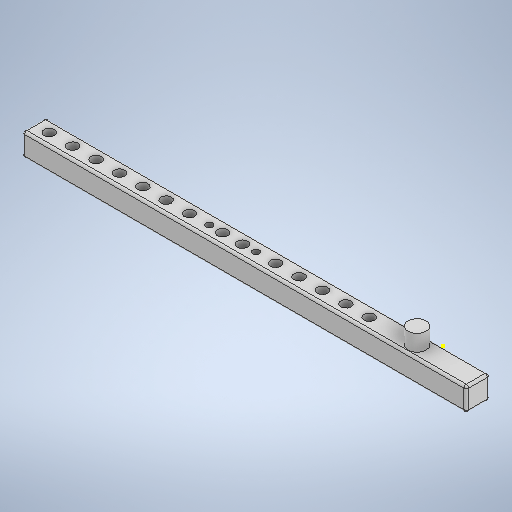
# Autodesk Inventor part: brazo apoyo
Saved by Autodesk Inventor 2025.2 (Build 292293000, 293)
## iProperties
Created: 2025-03-30
Part Number: brazo apoyo
Material: Generic
Document SubType Name: Modeling
Designer: maqmat
Density: 1 g/cm^3
Appearance: Default
Author: maqmat
Autodesk Inventor part; units mm, degrees
ref_plane "YZ Plane" through (0, 0, 0) normal (1, 0, 0) x (0, 1, 0)
ref_plane "XZ Plane" through (0, 0, 0) normal (0, 1, 0) x (-1, 0, 0)
ref_plane "XY Plane" through (0, 0, 0) normal (0, 0, 1) x (1, 0, 0)
sketch "Sketch1" plane through (0, 0, 0) normal (0, 1, 0) x (-1, 0, 0)
  line L0 (0, 0) -> (170, 0)
  line L1 (170, 0) -> (170, 10)
  line L2 (170, 10) -> (0, 10)
  line L3 (0, 10) -> (0, 0)
  dimension "d0" = 170
  dimension "d1" = 10
  constraints: 8 end point, 2 parallel, 1 horizontal, 1 perpendicular
  measures "d0" distance of L2.end L1.end
  measures "d1" distance of L1.end L0.end
extrude "Extrusion1" add sketch "Sketch1" along normal blind 10
sketch "Sketch2" plane through (0, 10, 0) normal (0, 1, 0) x (1, 0, 0)
  line L0 (0, -10) -> (0, 0) projected
  line L1 (0, -5) -> (-2.2, -5)
  circle A0 centre (-6.1, -5) radius 3.9
  line L2 (0, 0) -> (-170, 0) projected
  line L3 (-170, -10) -> (0, -10) projected
  circle A1 centre (-75, -5) radius 1.5
  circle A2 centre (-95, -5) radius 1.5
  dimension "d35" = 10
  dimension "d4" = 2.2
  dimension "d8" = 3
  dimension "d9" = 3
  constraints: 2 centre point, 2 end point, 1 horizontal, 1 horizontal alignment, 1 midpoint, 2 other
  measures "d4" distance of L1.start L1.end
  measures "d8" diameter of A1
  measures "d9" diameter of A2
extrude "Extrusion2" cut sketch "Sketch2" against normal blind 10 contours A1
extrude "Extrusion3" cut sketch "Sketch2" against normal blind 10 contours A2
extrude "Extrusion4" add sketch "Sketch2" along normal blind 7 contours A0
sketch "Sketch3" plane through (0, 10, 0) normal (0, 1, 0) x (1, 0, 0)
  line L0 (-170, 0) -> (-170, -10) projected
  line L1 (-170, -5) -> (-10, -5)
  circle A0 centre (-6.1, -5) radius 3.9 projected
  line L2 (-165.7, -5) -> (-163.45, -5)
  circle A1 centre (-163.45, -5) radius 2.25
  circle A2 centre (-153.45, -5) radius 2.25
  circle A3 centre (-143.45, -5) radius 2.25
  circle A4 centre (-133.45, -5) radius 2.25
  circle A5 centre (-123.45, -5) radius 2.25
  circle A6 centre (-113.45, -5) radius 2.25
  circle A7 centre (-103.45, -5) radius 2.25
  circle A8 centre (-95, -5) radius 1.5 projected
  line L3 (-93.5, -5) -> (-93.5, -7.9104)
  circle A9 centre (-75, -5) radius 1.5 projected
  line L4 (-76.5, -5) -> (-76.5, -7.25)
  line L5 (-93.5, -5) -> (-76.5, -5)
  line L6 (-85, -5) -> (-93.5, -5)
  line L7 (-85, -5) -> (-76.5, -5)
  circle A10 centre (-80.75, -5) radius 2.25
  circle A11 centre (-89.25, -5) radius 2.25
  line L8 (-10, -5) -> (-12, -5)
  line L9 (-10, -5) -> (-14.3, -5)
  line L10 (-14.3, -5) -> (-16.55, -5)
  circle A12 centre (-16.55, -5) radius 2.25
  circle A13 centre (-26.55, -5) radius 2.25
  circle A14 centre (-36.55, -5) radius 2.25
  circle A15 centre (-46.55, -5) radius 2.25
  circle A16 centre (-56.55, -5) radius 2.25
  circle A17 centre (-66.55, -5) radius 2.25
  point P0 (0, 0)
  point P1 (-155.7, -5)
  point P2 (-145.7, -5)
  point P3 (-135.7, -5)
  point P4 (-125.7, -5)
  point P5 (-115.7, -5)
  point P6 (-105.7, -5)
  point P7 (-24.3, -5)
  point P8 (-34.3, -5)
  point P9 (-44.3, -5)
  point P10 (-54.3, -5)
  point P11 (-64.3, -5)
  dimension "d20" = 10
  dimension "d32" = 10
  constraints: 38 horizontal alignment, 18 end point, 4 midpoint, 4 vertical, 3 horizontal, 2 centre point, 2 coincident, 39 other
  measures "d20" distance of point (-163.45, -5) point (-153.45, -5)
  measures "d32" distance of point (-16.55, -5) point (-26.55, -5)
extrude "Extrusion5" cut sketch "Sketch3" against normal blind 10 contours A1 L1 | L1 A1 | L1 A12 | L1 A12 | A2 L1 | L1 A2 | A3 L1 | L1 A3 | A4 L1 | L1 A4 | A5 L1 | L1 A5 | A6 L1 | L1 A6 | A7 L1 | L1 A7 | A11 L1 | L1 A11 | A10 L1 | L1 A10 | A17 L1 | L1 A17 | A16 L1 | L1 A16 | A15 L1 | L1 A15 | A14 L1 | L1 A14 | A13 L1 | L1 A13
thread "Thread1" size "M3x0.5" class "6H" standard "ANSI Metric M Profile" full length
thread "Thread2" size "M3x0.5" class "6H" standard "ANSI Metric M Profile" full length
sketch "Sketch4" plane through (0, 10, 0) normal (0, 1, 0) x (1, 0, 0)
  circle A0 centre (-16.55, -5) radius 2.25 projected
  circle A1 centre (-16.55, -5) radius 2.25
  point P0 (0, 0)
  constraints: 1 centre point, 1 coincident
extrude "Extrusion6" add sketch "Sketch4" against normal blind 10
sketch "Sketch5" plane through (0, 0, 10) normal (1, 0, 0) x (0, 0, -1)
  line L0 (10, 0) -> (0, 0) projected
  line L1 (0, 0) -> (0, 10) projected
  line L2 (10, 0) -> (0, 0)
  line L3 (0, 0) -> (0, 10)
  line L4 (0, 10) -> (10, 10)
  line L5 (10, 10) -> (10, 0)
  constraints: 8 end point, 2 parallel, 1 horizontal, 1 perpendicular
extrude "Extrusion7" add sketch "Sketch5" along normal blind 10
sketch "Sketch6" plane through (10, 0, 10) normal (1, 0, 0) x (0, 0, -1)
  line L0 (0, 0) -> (10, 0) projected
  line L1 (0, 10) -> (0, 0) projected
  line L2 (10, 0) -> (0, 0)
  line L3 (0, 0) -> (0, 10)
  line L4 (0, 10) -> (10, 10)
  line L5 (10, 10) -> (10, 0)
  constraints: 8 end point, 2 parallel, 1 horizontal, 1 perpendicular
extrude "Extrusion8" add sketch "Sketch6" along normal blind 10
sketch "Sketch7" plane through (0, 10, 0) normal (0, 1, 0) x (1, 0, 0)
  point P0 (0, 0)
fillet "Fillet3" radius 1 11 edges at (-75, 10, 10) (-75, 0, 10) (-75, 10, 0) (20, 5, 10) (20, 5, 0) (20, 0, 5) (-170, 10, 5) (-170, 5, 10) (-170, 5, 0) (-170, 0, 5) (-75, 0, 0)
fillet "Fillet4" radius 1 3 edges at (19.7071, 9.7071, 9.7071) (19.7071, 9.7071, 0.2929) (20, 10, 5)
body "Solid1"
